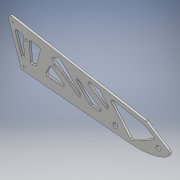
# Autodesk Inventor part: bracket
Saved by Autodesk Inventor 2018.3 (Build 223284000, 284)
## iProperties
Created: 2018-06-13
Part Number: bracket
Material: 一般
Document SubType Name: Modeling
Designer: ku_sk
Density: 1 g/cm^3
Appearance: 既定
Author: ku_sk
Autodesk Inventor part; units mm, degrees
ref_plane "YZ Plane" through (0, 0, 0) normal (1, 0, 0) x (0, 1, 0)
ref_plane "XZ Plane" through (0, 0, 0) normal (0, 1, 0) x (-1, 0, 0)
ref_plane "XY Plane" through (0, 0, 0) normal (0, 0, 1) x (1, 0, 0)
sketch "スケッチ1" plane through (0, 0, 0) normal (0, 1, 0) x (-1, 0, 0)
  arc A0 (219.4609, 18.684) -> (224.588, 12.5827) centre (222.2914, 15.8576) ccw projected
  line L0 (224.588, 12.5827) -> (289.8158, 58.3257) projected
  arc A1 (289.8158, 58.3257) -> (289.207, 65.2271) centre (287.5191, 61.6007) ccw projected
  line L1 (289.207, 65.2271) -> (275.8597, 71.4394) projected
  arc A2 (275.8597, 71.4394) -> (271.3414, 70.6393) centre (274.1718, 67.8129) ccw projected
  line L2 (271.3414, 70.6393) -> (219.4609, 18.684) projected
  arc A3 (192.5589, 7.22) -> (195.0379, 8.3782) centre (192.2074, 11.2045) ccw projected
  line L3 (195.0379, 8.3782) -> (228.7404, 42.1292) projected
  arc A4 (228.7404, 42.1292) -> (223.7337, 48.3118) centre (225.9099, 44.9556) ccw projected
  line L4 (223.7337, 48.3118) -> (168.7921, 12.6873) projected
  arc A5 (168.7921, 12.6873) -> (171.3198, 5.3465) centre (170.9683, 9.3311) ccw projected
  line L5 (171.3198, 5.3465) -> (192.5589, 7.22) projected
  arc A6 (303.5017, 17.0062) -> (306.7742, 22.6838) centre (303.1502, 20.9907) ccw projected
  line L6 (306.7742, 22.6838) -> (298.5118, 40.3693) projected
  arc A7 (298.5118, 40.3693) -> (292.5912, 41.9512) centre (294.8878, 38.6762) ccw projected
  line L7 (292.5912, 41.9512) -> (262.555, 20.8874) projected
  arc A8 (262.555, 20.8874) -> (265.2032, 13.6279) centre (264.8517, 17.6124) ccw projected
  line L8 (265.2032, 13.6279) -> (303.5017, 17.0062) projected
  arc A9 (368.602, 77.1527) -> (365.3028, 73.4818) centre (369.2938, 73.2129) ccw projected
  line L9 (365.3028, 73.4818) -> (362.3615, 29.8254) projected
  arc A10 (362.3615, 29.8254) -> (370.1378, 28.2638) centre (366.3525, 29.5565) ccw projected
  line L10 (370.1378, 28.2638) -> (385.8094, 74.1557) projected
  arc A11 (385.8094, 74.1557) -> (381.3322, 79.3881) centre (382.024, 75.4484) ccw projected
  line L11 (381.3322, 79.3881) -> (368.602, 77.1527) projected
  arc A12 (148.799, 26.9271) -> (154.0376, 20.9976) centre (151.8614, 24.3538) ccw projected
  line L12 (154.0376, 20.9976) -> (198.0951, 49.5648) projected
  arc A13 (198.0951, 49.5648) -> (195.2271, 56.8608) centre (195.9189, 52.921) ccw projected
  line L13 (195.2271, 56.8608) -> (171.7035, 52.73) projected
  arc A14 (171.7035, 52.73) -> (169.333, 51.3636) centre (172.3953, 48.7903) ccw projected
  line L14 (169.333, 51.3636) -> (148.799, 26.9271) projected
  arc A15 (342.152, 22.8457) -> (347.1008, 26.4604) centre (343.1098, 26.7293) ccw projected
  line L15 (347.1008, 26.4604) -> (349.9566, 68.8476) projected
  arc A16 (349.9566, 68.8476) -> (345.2738, 73.0562) centre (345.9657, 69.1165) ccw projected
  line L16 (345.2738, 73.0562) -> (324.8488, 69.4695) projected
  arc A17 (324.8488, 69.4695) -> (321.6761, 64.4972) centre (325.5406, 65.5298) ccw projected
  line L17 (321.6761, 64.4972) -> (331.5354, 27.5983) projected
  arc A18 (331.5354, 27.5983) -> (334.442, 24.7472) centre (335.3998, 28.6309) ccw projected
  line L18 (334.442, 24.7472) -> (342.152, 22.8457) projected
  arc A19 (87.3543, -17.9583) -> (92.2946, -16.9998) centre (89.2322, -14.4265) ccw projected
  line L19 (92.2946, -16.9998) -> (140.2153, 40.0283) projected
  arc A20 (140.2153, 40.0283) -> (136.4611, 46.5414) centre (137.1529, 42.6016) ccw projected
  line L20 (136.4611, 46.5414) -> (57.1601, 32.616) projected
  arc A21 (57.1601, 32.616) -> (55.7323, 32.0685) centre (57.852, 28.6763) ccw projected
  line L21 (55.7323, 32.0685) -> (32.8911, 17.7957) projected
  arc A22 (32.8911, 17.7957) -> (33.1329, 10.8717) centre (35.0108, 14.4035) ccw projected
  line L22 (33.1329, 10.8717) -> (87.3543, -17.9583) projected
  circle A23 centre (362.9417, 7.1911) radius 2.5 projected
  circle A24 centre (391.6841, 91.3589) radius 2.5 projected
  circle A25 centre (20.1088, -0.8575) radius 6 projected
  circle A26 centre (130.7072, -5.574) radius 6 projected
  arc A27 (402.7873, 92.9292) -> (394.9522, 102.0858) centre (396.1629, 95.1913) ccw projected
  line L23 (371.564, 1.4963) -> (402.7873, 92.9292) projected
  arc A28 (366.4132, -2.5415) -> (371.564, 1.4963) centre (365.886, 3.4353) ccw projected
  line L24 (101.4688, -25.912) -> (366.4132, -2.5415) projected
  arc A29 (75.9435, -27.404) -> (101.4688, -25.912) centre (63.5115, 404.3974) ccw projected
  arc A30 (28.9907, -22.4032) -> (75.9435, -27.404) centre (70.8911, 148.0818) ccw projected
  arc A31 (1.6336, -11.2619) -> (28.9907, -22.4032) centre (53.2618, 76.3513) ccw projected
  arc A32 (-5.8527, -4.9449) -> (1.6336, -11.2619) centre (16.4695, 13.9147) ccw projected
  arc A33 (-4.0602, 6.4977) -> (-5.8527, -4.9449) centre (0, 0) ccw projected
  line L25 (51.7543, 41.3745) -> (-4.0602, 6.4977) projected
  arc A34 (53.8961, 42.1958) -> (51.7543, 41.3745) centre (54.9338, 36.2863) ccw projected
  line L26 (394.9522, 102.0858) -> (53.8961, 42.1958) projected
  circle A35 centre (285.7217, 47.1567) radius 3 projected
  circle A36 centre (357.6123, 68.7377) radius 3 projected
  point P0 (0, 0)
extrude "押し出し1" add sketch "スケッチ1" along normal mid plane 5
